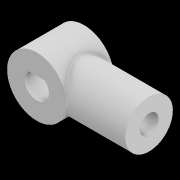
# Autodesk Inventor part: pieza para aplicar torque en la salida de la caja reductora
Saved by Autodesk Inventor 2020 (Build 240168000, 168)
## iProperties
Created: 2021-11-05
Part Number: pieza para aplicar torque en la salida de la caja reductora
Material: Generic
Document SubType Name: Modeling
Designer: juan
Density: 1 g/cm^3
Appearance: Default
Author: juan
Autodesk Inventor part; units mm, degrees
ref_plane "XZ Plane" through (0, 0, 0) normal (0, 1, 0) x (-1, 0, 0)
ref_plane "XY Plane" through (0, 0, 0) normal (0, 0, 1) x (1, 0, 0)
sketch "Sketch1" plane through (0, 0, 0) normal (0, 0, 1) x (1, 0, 0)
  arc A0 (-1.3416, 1.55) -> (1.3416, 1.55) centre (0, 0) ccw
  circle A1 centre (0, 0) radius 5
  line L0 (-1.3416, 1.55) -> (1.3416, 1.55)
  dimension "d0" = 4.1
  dimension "d2" = 0.5
  dimension "d17" = 10
  constraints: 2 centre point, 2 coincident, 2 end point, 2 point on circle, 1 horizontal
  measures "d0" diameter of A0
  measures "d2" distance edge to line of A0 L0
  measures "d17" diameter of A1
extrude "Extrusion1" add sketch "Sketch1" along normal blind 8
ref_plane "Work Plane1" through (5, 0, 0) normal (1, 0, 0) x (0, 1, 0)
sketch "Sketch2" plane through (5, 0, 0) normal (1, 0, 0) x (0, 1, 0)
  line L0 (5, 8) -> (-5, 8) construction
  line L1 (5, 0) -> (-5, 0) construction
  line L2 (5, 0) -> (5, 8) construction
  line L3 (-5, 0) -> (-5, 8) construction
  circle A0 centre (0, 4) radius 4
  point P0 (0, 0)
  point P1 (0, 0)
  point P2 (5, 4)
  dimension "d5" = 8
  constraints: 2 midpoint, 1 centre point, 1 horizontal alignment, 1 vertical alignment
  measures "d5" diameter of A0
extrude "Extrusion2" add sketch "Sketch2" along normal blind 10 and the other way blind 2
sketch "Sketch3" plane through (15, 0, 4) normal (1, 0, 0) x (0, 0, -1)
  point P0 (4, 0)
  point P1 (0, 0)
hole "Hole1" at (15, 0, 4) direction (-1, 0, 0) diameter 3.2 depth 10
fillet "Fillet1" radius 0.5 4 edges at (3.9799, 3.0266, 1.3847) (3.9799, 3.0266, 6.6153) (3.9794, -3.0272, 1.3855) (3.9799, -3.0266, 6.6153)
body "Solid1"
